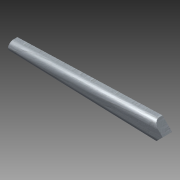
# Autodesk Inventor part: Lift_Support
Saved by Autodesk Inventor 2011 SP1 (Build 150282100, 282)
## iProperties
Created: 2011-06-11
Part Number: Lift_Support
Document SubType Name: Modeling
Designer: Andrew G. Meyer
Mass: 5.50305 g
Surface Area: 29.8003 cm^2
Volume: 5.50305 cm^3
Density: 1 g/cm^3
Author: Andrew G. Meyer
Autodesk Inventor part; units mm, degrees
ref_plane "YZ Plane" through (0, 0, 0) normal (1, 0, 0) x (0, 1, 0)
ref_plane "XZ Plane" through (0, 0, 0) normal (0, 1, 0) x (-1, 0, 0)
ref_plane "XY Plane" through (0, 0, 0) normal (0, 0, 1) x (1, 0, 0)
sketch "Sketch1" plane through (0, 0, 0) normal (0, 0, 1) x (1, 0, 0)
  line L0 (0, 0) -> (-6.35, 6.35)
  line L1 (-6.35, 6.35) -> (-103.1386, 3.175)
  line L2 (0, 0) -> (-6.35, -6.35)
  line L3 (-6.35, -6.35) -> (-103.1386, -3.175)
  arc A0 (-103.1386, 3.175) -> (-103.1386, -3.175) centre (0, 0) ccw
  line L4 (0, 0) -> (24.3963, 0) construction
  dimension "d0" = 103.1875
  dimension "d1" = 6.35
  dimension "d2" = 6.35
  dimension "d8" = 135
  constraints: 11 end point, 2 equal length, 2 point on circle, 1 centre point, 1 coincident, 1 horizontal, 1 perpendicular
  measures "d0" radius of A0
  measures "d1" distance of L3.end L1.end
  measures "d2" horizontal distance of L0.start L0.end
  measures "d8" angle of L0 L4
extrude "Extrusion1" add sketch "Sketch1" along normal blind 6.35
fillet "Fillet1" radius 3.81 2 edges at (-54.7443, -4.7625, 6.35) (-54.7443, 4.7625, 6.35)
body "Solid1"
